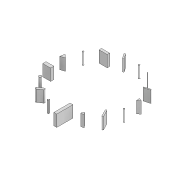
# Autodesk Inventor part: simple_ring2
Saved by Autodesk Inventor 2021 (Build 250183000, 183)
## iProperties
Created: 2022-04-12
Part Number: simple_ring2
Material: Generic
Document SubType Name: Modeling
Designer: Derm
Density: 1 g/cm^3
Appearance: Default
Author: Derm
Autodesk Inventor part; units mm, degrees
ref_plane "YZ Plane" through (0, 0, 0) normal (1, 0, 0) x (0, 1, 0)
ref_plane "XZ Plane" through (0, 0, 0) normal (0, 1, 0) x (-1, 0, 0)
ref_plane "XY Plane" through (0, 0, 0) normal (0, 0, 1) x (1, 0, 0)
sketch "Sketch1" plane through (0, 0, 0) normal (0, 1, 0) x (-1, 0, 0)
  circle A0 centre (0, 0) radius 10000 construction
  line L0 (0, 0) -> (10000, 0)
  line L1 (0, 0) -> (9807.8528, -1950.9032) construction
  circle A1 centre (8314.6961, 5555.7023) radius 346.929
  circle A2 centre (8314.6961, -5555.7023) radius 187.6046
  circle A3 centre (-9807.8528, 1950.9032) radius 174.621
  circle A4 centre (-1950.9032, -9807.8528) radius 192.1472
  line L2 (10829.2054, 1528.2394) -> (8786.5002, 1528.2394)
  line L3 (8786.5002, 1528.2394) -> (8786.5002, 2373.5671)
  line L4 (8786.5002, 2373.5671) -> (10829.2054, 2373.5671)
  line L5 (10829.2054, 2373.5671) -> (10829.2054, 1528.2394)
  line L6 (10829.2054, 1528.2394) -> (8786.5002, 2373.5671) construction
  line L7 (8786.5002, 1528.2394) -> (10829.2054, 2373.5671) construction
  line L8 (6618.1197, -8628.5526) -> (4493.285, -8628.5526)
  line L9 (4493.285, -8628.5526) -> (4493.285, -8000.8397)
  line L10 (4493.285, -8000.8397) -> (6618.1197, -8000.8397)
  line L11 (6618.1197, -8000.8397) -> (6618.1197, -8628.5526)
  line L12 (6618.1197, -8628.5526) -> (4493.285, -8000.8397) construction
  line L13 (4493.285, -8628.5526) -> (6618.1197, -8000.8397) construction
  line L14 (-1574.432, 11914.1393) -> (-2327.3745, 11914.1393)
  line L15 (-2327.3745, 11914.1393) -> (-2327.3745, 7701.5663)
  line L16 (-2327.3745, 7701.5663) -> (-1574.432, 7701.5663)
  line L17 (-1574.432, 7701.5663) -> (-1574.432, 11914.1393)
  line L18 (-1574.432, 11914.1393) -> (-2327.3745, 7701.5663) construction
  line L19 (-2327.3745, 11914.1393) -> (-1574.432, 7701.5663) construction
  line L20 (6111.4047, 8698.8883) -> (5000, 7930.504) construction
  line L21 (5957.5036, 8921.4935) -> (4846.0989, 8153.1092)
  line L22 (5153.9011, 7707.8988) -> (6265.3057, 8476.283)
  arc A5 (6265.3057, 8476.283) -> (5957.5036, 8921.4935) centre (6111.4047, 8698.8883) ccw
  arc A6 (4846.0989, 8153.1092) -> (5153.9011, 7707.8988) centre (5000, 7930.504) ccw
  line L23 (1569.0875, -9255.5877) -> (2332.719, -10360.1179) construction
  line L24 (1438.3811, -9345.9533) -> (2202.0126, -10450.4835)
  line L25 (2463.4253, -10269.7523) -> (1699.7938, -9165.2221)
  arc A7 (1699.7938, -9165.2221) -> (1438.3811, -9345.9533) centre (1569.0875, -9255.5877) ccw
  arc A8 (2202.0126, -10450.4835) -> (2463.4253, -10269.7523) centre (2332.719, -10360.1179) ccw
  line L26 (-6411.4053, -7464.1701) -> (-4699.9994, -9165.2221) construction
  line L27 (-6390.7191, -7443.358) -> (-4679.3132, -9144.41)
  line L28 (-4720.6856, -9186.0343) -> (-6432.0915, -7484.9822)
  arc A9 (-6390.7191, -7443.358) -> (-6432.0915, -7484.9822) centre (-6411.4053, -7464.1701) ccw
  arc A10 (-4720.6856, -9186.0343) -> (-4679.3132, -9144.41) centre (-4699.9994, -9165.2221) ccw
  line L29 (-7627.8496, -5368.0977) -> (-9001.5427, -5743.3069) construction
  line L30 (-7662.5032, -5241.2261) -> (-9036.1963, -5616.4353)
  line L31 (-8966.8891, -5870.1786) -> (-7593.196, -5494.9694)
  arc A11 (-7593.196, -5494.9694) -> (-7662.5032, -5241.2261) centre (-7627.8496, -5368.0977) ccw
  arc A12 (-9036.1963, -5616.4353) -> (-8966.8891, -5870.1786) centre (-9001.5427, -5743.3069) ccw
  line L32 (-8745.7152, 6414.9242) -> (-7883.677, 4696.4804) construction
  line L33 (-8898.4171, 6338.323) -> (-8036.3789, 4619.8792)
  line L34 (-7730.9752, 4773.0816) -> (-8593.0134, 6491.5254)
  arc A13 (-8593.0134, 6491.5254) -> (-8898.4171, 6338.323) centre (-8745.7152, 6414.9242) ccw
  arc A14 (-8036.3789, 4619.8792) -> (-7730.9752, 4773.0816) centre (-7883.677, 4696.4804) ccw
  line L35 (1820.1969, 9564.3207) -> (1805.3514, 10042.8139)
  line L36 (1805.3514, 10042.8139) -> (2227.1614, 9816.4238)
  line L37 (2227.1614, 9816.4238) -> (1820.1969, 9564.3207)
  line L38 (9154.6321, -1820.9695) -> (10246.989, -1450.1643)
  line L39 (10246.989, -1450.1643) -> (10021.9373, -2581.5758)
  line L40 (10021.9373, -2581.5758) -> (9154.6321, -1820.9695)
  line L41 (-5960.5026, 8476.283) -> (-5213.3638, 8584.47)
  line L42 (-5213.3638, 8584.47) -> (-5493.2406, 7883.3354)
  line L43 (-5493.2406, 7883.3354) -> (-5960.5026, 8476.283)
  line L44 (-10298.5617, -2015.8701) -> (-9618.7613, -1493.4535)
  line L45 (-9618.7613, -1493.4535) -> (-9506.2354, -2343.3861)
  line L46 (-9506.2354, -2343.3861) -> (-10298.5617, -2015.8701)
  point P0 (9807.8528, 1950.9032)
  point P1 (5555.7023, 8314.6961)
  point P2 (1950.9032, 9807.8528)
  point P3 (-1950.9032, 9807.8528)
  point P4 (-5555.7023, 8314.6961)
  point P5 (-8314.6961, 5555.7023)
  point P6 (-9807.8528, -1950.9032)
  point P7 (-8314.6961, -5555.7023)
  point P8 (-5555.7023, -8314.6961)
  point P9 (1950.9032, -9807.8528)
  point P10 (5555.7023, -8314.6961)
  point P11 (1950.9032, 9807.8528)
  point P12 (-5555.7023, 8314.6961)
  point P13 (-9807.8528, -1950.9032)
  dimension "d0" = 20000
  dimension "d1" = 11.25
  dimension "d4" = 360
  constraints: 104 end point, 22 point on circle, 20 tangent, 15 centre point, 11 midpoint, 11 parallel, 10 coincident, 4 horizontal, 4 perpendicular, 2 point on line, 45 other
  measures "d0" diameter of A0
  measures "d1" angle of L1 L0
extrude "Extrusion1" add sketch "Sketch1" along normal mid plane 3000
body "Solid1"
